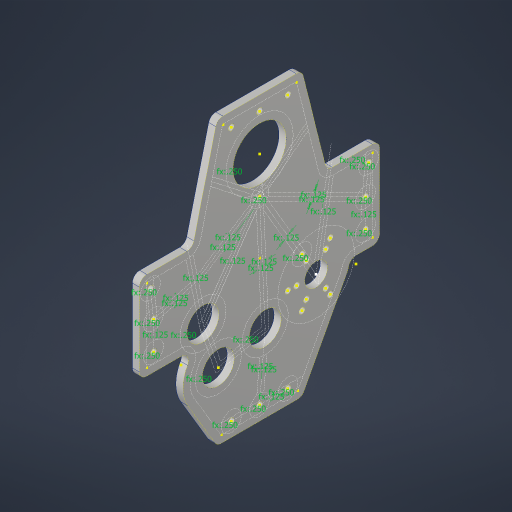
# Autodesk Inventor part: EL2-CGB-001
Saved by Autodesk Inventor 2023.4 (Build 274418000, 418)
## iProperties
Created: 2025-01-19
Part Number: EL2-CGB-001
Material: Aluminum 6061
Document SubType Name: Modeling
Designer: mavericks
Density: 2.7 g/cm^3
Appearance: Aluminum - Flat
Author: mavericks
Autodesk Inventor part; units mm, degrees
ref_plane "YZ Plane" through (0, 0, 0) normal (1, 0, 0) x (0, 1, 0)
ref_plane "XZ Plane" through (0, 0, 0) normal (0, 1, 0) x (-1, 0, 0)
ref_plane "XY Plane" through (0, 0, 0) normal (0, 0, 1) x (1, 0, 0)
sketch "Sketch1" plane through (0, 0, 0) normal (1, 0, 0) x (0, 1, 0)
  line L0 (127, 107.95) -> (-127, 107.95) construction
  line L1 (-127, 107.95) -> (-127, 82.55) construction
  line L2 (-127, 82.55) -> (127, 82.55) construction
  line L3 (127, 82.55) -> (127, 107.95) construction
  line L4 (-44.45, 128.7526) -> (-69.85, 128.7526) construction
  line L5 (-69.85, 128.7526) -> (-69.85, 79.4258) construction
  line L6 (-69.85, 79.4258) -> (-44.45, 79.4258) construction
  line L7 (-44.45, 79.4258) -> (-44.45, 128.7526) construction
  line L8 (69.85, 128.7526) -> (44.45, 128.7526) construction
  line L9 (44.45, 128.7526) -> (44.45, 79.4258) construction
  line L10 (44.45, 79.4258) -> (69.85, 79.4258) construction
  line L11 (69.85, 79.4258) -> (69.85, 128.7526) construction
  line L12 (44.45, 104.0892) -> (-44.45, 104.0892) construction
  line L13 (0, 0) -> (-27.2932, 0) construction
  line L14 (127, -107.95) -> (-127, -107.95) construction
  line L15 (-127, -107.95) -> (-127, -82.55) construction
  line L16 (-127, -82.55) -> (127, -82.55) construction
  line L17 (127, -82.55) -> (127, -107.95) construction
  line L18 (-44.45, -128.7526) -> (-69.85, -128.7526) construction
  line L19 (-69.85, -128.7526) -> (-69.85, -79.4258) construction
  line L20 (-69.85, -79.4258) -> (-44.45, -79.4258) construction
  line L21 (-44.45, -79.4258) -> (-44.45, -128.7526) construction
  line L22 (69.85, -128.7526) -> (44.45, -128.7526) construction
  line L23 (44.45, -128.7526) -> (44.45, -79.4258) construction
  line L24 (44.45, -79.4258) -> (69.85, -79.4258) construction
  line L25 (69.85, -79.4258) -> (69.85, -128.7526) construction
  line L26 (44.45, -104.0892) -> (-44.45, -104.0892) construction
  line L27 (127, 82.55) -> (101.6, 82.55) construction
  line L28 (101.6, 82.55) -> (101.6, -82.55) construction
  line L29 (101.6, -82.55) -> (127, -82.55) construction
  line L30 (127, -82.55) -> (127, 82.55) construction
  line L31 (-127, 82.55) -> (-101.6, 82.55) construction
  line L32 (-101.6, 82.55) -> (-101.6, -82.55) construction
  line L33 (-101.6, -82.55) -> (-127, -82.55) construction
  line L34 (-127, -82.55) -> (-127, 82.55) construction
  point P0 (0, 82.55)
  point P1 (0, 104.0892)
  point P2 (0, -82.55)
  point P3 (0, -104.0892)
  dimension "d0" = 254
  dimension "d1" = 25.4
  dimension "d2" = 82.55
  dimension "d3" = 25.4
  dimension "d4" = 49.3268
  dimension "d6" = 88.9
  dimension "d7" = 3.1242
  dimension "d8" = 25.4
  dimension "d9" = 25.4
  constraints: 70 end point, 16 symmetric about line, 12 parallel, 7 horizontal, 5 perpendicular, 4 midpoint, 2 vertical alignment, 1 horizontal alignment, 1 point on line
  measures "d0" distance of L2.end L1.end
  measures "d1" distance of L1.end L0.end
  measures "d2" vertical distance of L13.start L2.end
  measures "d3" distance of L6.end L5.end
  measures "d4" distance of L5.end L4.end
  measures "d6" distance of L4.start L8.end
  measures "d7" distance from line of L2 L6.end
  measures "d8" distance between parallel lines of L28 L30
  measures "d9" distance between parallel lines of L34 L32
sketch "Sketch2" plane through (0, 0, 0) normal (1, 0, 0) x (0, 1, 0)
  line L0 (-127, 107.95) -> (-127, 82.55) construction
  line L1 (44.45, 104.0892) -> (-44.45, 104.0892) construction
  line L2 (-127, 82.55) -> (127, 82.55) construction
  line L3 (127, 107.95) -> (-127, 107.95) construction
  line L4 (44.45, 79.4258) -> (69.85, 79.4258) construction
  line L5 (127, 82.55) -> (127, 107.95) construction
  line L6 (-69.85, 79.4258) -> (-44.45, 79.4258) construction
  line L7 (-44.45, 79.4258) -> (-44.45, 128.7526) construction
  line L8 (-69.85, 128.7526) -> (-69.85, 79.4258) construction
  line L9 (-44.45, 128.7526) -> (-69.85, 128.7526) construction
  line L10 (101.6, 82.55) -> (101.6, -82.55) construction
  line L11 (127, -82.55) -> (127, 82.55) construction
  line L12 (-127, -82.55) -> (127, -82.55) construction
  line L13 (127, -107.95) -> (-127, -107.95) construction
  line L14 (44.45, -104.0892) -> (-44.45, -104.0892) construction
  line L15 (-127, 82.55) -> (-101.6, 82.55) construction
  line L16 (-101.6, 82.55) -> (-101.6, -82.55) construction
  line L17 (-127, -82.55) -> (-127, 82.55) construction
  line L18 (-69.85, -79.4258) -> (-44.45, -79.4258) construction
  line L19 (-101.6, -82.55) -> (-127, -82.55) construction
  line L20 (-44.45, -79.4258) -> (-44.45, -128.7526) construction
  line L21 (-44.45, -128.7526) -> (-69.85, -128.7526) construction
  line L22 (-69.85, -128.7526) -> (-69.85, -79.4258) construction
  line L23 (-127, -107.95) -> (-127, -82.55) construction
  line L24 (44.45, -79.4258) -> (69.85, -79.4258) construction
  line L25 (44.45, -128.7526) -> (44.45, -79.4258) construction
  line L26 (101.6, -82.55) -> (127, -82.55) construction
  line L27 (69.85, -128.7526) -> (44.45, -128.7526) construction
  line L28 (69.85, -79.4258) -> (69.85, -128.7526) construction
  line L29 (127, -82.55) -> (127, -107.95) construction
  line L30 (69.85, 128.7526) -> (44.45, 128.7526) construction
  line L31 (44.45, 128.7526) -> (44.45, 79.4258) construction
  line L32 (69.85, 79.4258) -> (69.85, 128.7526) construction
  line L33 (127, 82.55) -> (101.6, 82.55) construction
  circle A0 centre (-38.1, -50.8) radius 7.62 construction
  circle A1 centre (-57.15, -5.08) radius 41.91 construction
  circle A2 centre (-57.15, -5.08) radius 11.43 construction
  circle A3 centre (-66.675, 37.0363) radius 31.75 construction
  circle A4 centre (-66.675, 37.0363) radius 15.24 construction
  circle A5 centre (-25.7473, 50.8) radius 27.94 construction
  circle A6 centre (-38.1, -50.8) radius 30.48 construction
  circle A7 centre (-38.1, -50.8) radius 10.16
  circle A8 centre (-57.15, -5.08) radius 14.2875
  circle A9 centre (-66.675, 37.0363) radius 14.2875
  circle A10 centre (-25.7473, 50.8) radius 14.2875
  circle A11 centre (-25.7473, 50.8) radius 20.6375 construction
  circle A12 centre (-66.675, 37.0363) radius 20.6375 construction
  circle A13 centre (-57.15, -5.08) radius 20.6375 construction
  circle A14 centre (-38.1, -50.8) radius 17.4625 construction
  circle A15 centre (-38.1, -50.8) radius 25.4 construction
  line L34 (-41.275, -131.9276) -> (-41.275, -76.2508) construction
  line L35 (-41.275, -76.2508) -> (-73.025, -76.2508) construction
  line L36 (-73.025, -76.2508) -> (-73.025, -131.9276) construction
  line L37 (-73.025, -131.9276) -> (-41.275, -131.9276) construction
  line L38 (-52.3959, -77.7195) -> (-127, -38.1)
  line L39 (-127, -38.1) -> (-127, 38.1)
  line L40 (-127, 38.1) -> (-41.275, 38.1) construction
  line L41 (-41.275, 38.1) -> (-41.275, 104.0892) construction
  arc A16 (-52.3959, -77.7195) -> (-41.275, -81.1142) centre (-38.1, -50.8) ccw
  circle A17 centre (80.9686, 0) radius 23.8125
  circle A18 centre (80.9686, 0) radius 33.3375 construction
  line L42 (37.9487, 60.325) -> (127, 38.1)
  line L43 (127, 38.1) -> (127, -38.1)
  line L44 (127, -38.1) -> (37.9487, -60.325)
  line L45 (37.9487, -60.325) -> (37.9487, -107.95)
  line L46 (37.9487, -107.95) -> (-41.275, -107.95)
  line L47 (-41.275, -107.95) -> (-41.275, -81.1142)
  line L48 (37.9487, 60.325) -> (37.9487, 107.95)
  line L49 (37.9487, 107.95) -> (-41.275, 107.95)
  arc A19 (-23.3654, 68.8297) -> (-38.2397, 37.5831) centre (-25.7473, 50.8) ccw construction
  arc A20 (43.4827, -39.6598) -> (88.1161, 54.1018) centre (80.9686, 0) ccw construction
  line L50 (-41.275, 107.95) -> (-41.275, 56.0863)
  line L51 (-82.9044, 64.325) -> (-127, 38.1)
  arc A21 (-41.275, 56.0863) -> (-82.9044, 64.325) centre (-66.675, 37.0363) ccw
  line L52 (88.1161, 54.1018) -> (-23.3654, 68.8297) construction
  line L53 (43.4827, -39.6598) -> (-38.2397, 37.5831) construction
  circle A22 centre (80.9686, 0) radius 11.1125 construction
  point P0 (25.2487, 98.0186)
  point P1 (0, 95.25)
  point P2 (25.2487, -98.0186)
  point P3 (0, -95.25)
  point P4 (-25.4, -95.25)
  point P5 (-25.4, 95.25)
  point P6 (127, -95.25)
  point P7 (127, 95.25)
  point P8 (0, -82.55)
  point P9 (-114.3, 25.4)
  point P10 (-114.3, 0)
  point P11 (-114.3, -25.4)
  point P12 (-101.6, 0)
  point P13 (-114.3, 82.55)
  point P14 (-38.1, -25.4)
  point P15 (-38.1, -33.3375)
  point P16 (-60.097, -38.1)
  point P17 (-53.223, -42.0688)
  point P18 (-60.097, -63.5)
  point P19 (-53.223, -59.5312)
  point P20 (-38.1, -76.2)
  point P21 (-38.1, -68.2625)
  point P22 (-16.103, -63.5)
  point P23 (-22.977, -59.5313)
  point P24 (-16.103, -38.1)
  point P25 (-22.977, -42.0688)
  point P26 (44.45, 104.0892)
  point P27 (-127, 0)
  point P28 (-127, 0)
  point P29 (101.6, 0)
  point P30 (114.3, 25.4)
  point P31 (114.3, 0)
  point P32 (114.3, -25.4)
  point P33 (114.3, 82.55)
  point P34 (127, 0)
  point P35 (-41.275, -76.8809)
  dimension "d33" = 34.925
  dimension "d34" = 50.8
  dimension "ChainLinks" = 50
  dimension "d10" = 15.24
  dimension "d11" = 83.82
  dimension "d12" = 22.86
  dimension "d13" = 63.5
  dimension "d14" = 30.48
  dimension "d15" = 55.88
  dimension "d16" = 60.96
  dimension "d19" = 63.5
  dimension "d23" = 20.32
  dimension "d24" = 28.575
  dimension "d26" = 25.4
  dimension "d27" = 25.4
  dimension "d28" = 25.4
  dimension "d29" = 25.4
  dimension "d30" = 6.35
  dimension "d31" = 6.35
  dimension "d32" = 6.35
  dimension "d37" = 360
  dimension "d41" = 3.175
  dimension "d42" = 76.2
  dimension "d60" = 101.7513
  dimension "d63" = 31.75
  dimension "d64" = 44.45
  dimension "d66" = 34.925
  dimension "d67" = 31.75
  dimension "d68" = 47.625
  dimension "d70" = 9.525
  dimension "d71" = 47.625
  dimension "d73" = 118.1903
  dimension "d74" = 12.7
  dimension "d75" = 36.3728
  dimension "d76" = 109.1438
  dimension "d78" = 9.9314
  dimension "d79" = 9.9314
  dimension "d133" = 205.5979
  dimension "d134" = 45.7518
  dimension "d135" = 112.4501
  dimension "d141" = 22.225
  constraints: 40 end point, 21 centre point, 18 vertical alignment, 15 coincident, 12 point on circle, 11 horizontal alignment, 11 midpoint, 11 point on line, 9 tangent, 3 collinear, 2 equal radius, 2 perpendicular, 1 horizontal, 1 vertical, 20 other
  measures "d10" diameter of A0
  measures "d11" diameter of A1
  measures "d12" diameter of A2
  measures "d13" diameter of A3
  measures "d14" diameter of A4
  measures "d15" diameter of A5
  measures "d16" diameter of A6
  measures "d19" distance from line of L16 A0.centre
  measures "d23" diameter of A7
  measures "d24" diameter of A8
  measures "d26" distance of point (-25.4, 95.25) point (0, 95.25)
  measures "d27" distance of point (25.249, 98.019) point (0, 95.25)
  measures "d28" distance of point (-114.3, 0) point (-114.3, 25.4)
  measures "d29" distance of point (-114.3, 0) point (-114.3, -25.4)
  measures "d30" radial gap between concentric circles of A10 A11
  measures "d31" radial gap between concentric circles of A9 A12
  measures "d32" radial gap between concentric circles of A8 A13
  measures "d41" distance between parallel lines of L20 L34
  measures "d42" distance of L38.end L39.end
  measures "d60" distance from line of L5 point (25.249, 98.019)
  measures "d63" distance from line of L12 A0.centre
  measures "d64" distance from line of L16 A1.centre
  measures "d66" distance from line of L16 A3.centre
  measures "d67" distance from line of L2 A5.centre
  measures "d68" diameter of A17
  measures "d70" radial gap between concentric circles of A17 A18
  measures "d71" distance of L42.start L48.end
  measures "d73" distance of A17.centre A5.centre
  measures "d74" horizontal distance of point (25.249, 98.019) L48.end
  measures "d75" diameter of A19
  measures "d76" diameter of A20
  measures "d78" distance from line of point (25.249, 98.019) L3
  measures "d79" distance from line of L13 point (25.249, -98.019)
  measures "d135" distance of L52.start L52.end
  measures "d141" diameter of A22
extrude "Extrusion1" add sketch "Sketch2" along normal blind 6.35
hole "Mount Holes" at (0, -101.6, 82.55) at (0, -127, 107.95) at (0, -69.85, 79.4258) at (0, 44.45, -79.4258) at (0, 69.85, -79.4258) at (0, 44.45, -128.7526) at (0, 44.45, 128.7526) at (0, 25.2487, 98.0186) at (0, 0, 95.25) at (0, 25.2487, -98.0186) at (0, 0, -95.25) at (0, -25.4, -95.25) at (0, -25.4, 95.25) at (0, -114.3, 25.4) at (0, -114.3, 0) at (0, -114.3, -25.4) at (0, 114.3, 25.4) at (0, 114.3, 0) at (0, 114.3, -25.4) direction (1, 0, 0) diameter 5.1054 end through all clearance for "Flat Head Machine Screw (82)" size "#10" standard "Ansi Unified Screw Threads"
hole "Motor Mount Holes" at (0, -38.1, -33.3375) at (0, -60.097, -38.1) at (0, -53.223, -42.0688) at (0, -60.097, -63.5) at (0, -53.223, -59.5312) at (0, -16.103, -63.5) at (0, -22.977, -59.5313) at (0, -16.103, -38.1) at (0, -22.977, -42.0688) at (0, -38.1, -25.4) direction (1, 0, 0) diameter 5.1054 end through all clearance for "Flat Head Machine Screw (82)" size "#10" standard "Ansi Unified Screw Threads"
fillet "Fillet1" radius 6.604 12 edges at (3.175, -41.275, 107.95) (3.175, -127, 38.1) (3.175, -127, -38.1) (3.175, -41.275, -81.1142) (3.175, -41.275, -107.95) (3.175, 37.9487, -107.95) (3.175, 37.9487, -60.325) (3.175, 127, -38.1) (3.175, 127, 38.1) (3.175, 37.9487, 60.325) (3.175, 37.9487, 107.95) (3.175, -41.275, 56.0863)
sketch "Sketch8" plane through (6.35, 0, 0) normal (1, 0, 0) x (0, 0, -1)
  arc A0 (-107.95, -34.671) -> (-101.346, -41.275) centre (-101.346, -34.671) ccw projected
  line L0 (-107.95, -34.671) -> (-107.95, 31.3447) projected
  arc A1 (-101.346, 37.9487) -> (-107.95, 31.3447) centre (-101.346, 31.3447) ccw projected
  line L1 (-101.346, 37.9487) -> (-65.4834, 37.9487) projected
  arc A2 (-65.4834, 37.9487) -> (-59.0759, 42.9535) centre (-65.4834, 44.5527) ccw projected
  line L2 (-59.0759, 42.9535) -> (-39.3491, 121.9951) projected
  arc A3 (-32.9416, 127) -> (-39.3491, 121.9951) centre (-32.9416, 120.396) ccw projected
  line L3 (-32.9416, 127) -> (32.9416, 127) projected
  arc A4 (39.3491, 121.9951) -> (32.9416, 127) centre (32.9416, 120.396) ccw projected
  line L4 (39.3491, 121.9951) -> (59.0759, 42.9535) projected
  arc A5 (59.0759, 42.9535) -> (65.4834, 37.9487) centre (65.4834, 44.5527) ccw projected
  line L5 (65.4834, 37.9487) -> (101.346, 37.9487) projected
  arc A6 (107.95, 31.3447) -> (101.346, 37.9487) centre (101.346, 31.3447) ccw projected
  line L6 (107.95, 31.3447) -> (107.95, -34.671) projected
  arc A7 (101.346, -41.275) -> (107.95, -34.671) centre (101.346, -34.671) ccw projected
  line L7 (101.346, -41.275) -> (86.5714, -41.275) projected
  arc A8 (86.5714, -41.275) -> (80.2012, -46.1375) centre (86.5714, -47.879) ccw projected
  arc A9 (77.7195, -52.3959) -> (80.2012, -46.1375) centre (50.8, -38.1) ccw projected
  line L8 (77.7195, -52.3959) -> (39.9622, -123.4934) projected
  arc A10 (34.1297, -127) -> (39.9622, -123.4934) centre (34.1297, -120.396) ccw projected
  line L9 (34.1297, -127) -> (-34.3439, -127) projected
  arc A11 (-40.02, -123.7717) -> (-34.3439, -127) centre (-34.3439, -120.396) ccw projected
  line L10 (-40.02, -123.7717) -> (-64.325, -82.9044) projected
  arc A12 (-64.7124, -51.1154) -> (-64.325, -82.9044) centre (-37.0363, -66.675) ccw projected
  arc A13 (-64.7124, -51.1154) -> (-70.469, -41.275) centre (-70.469, -47.879) ccw projected
  line L11 (-70.469, -41.275) -> (-101.346, -41.275) projected
  circle A14 centre (42.0688, -22.977) radius 2.5527 projected
  circle A15 centre (59.5313, -22.977) radius 2.5527 projected
  circle A16 centre (59.5312, -53.223) radius 2.5527 projected
  circle A17 centre (42.0688, -53.223) radius 2.5527 projected
  circle A18 centre (33.3375, -38.1) radius 2.5527 projected
  circle A19 centre (38.1, -60.097) radius 2.5527 projected
  circle A20 centre (63.5, -60.097) radius 2.5527 projected
  circle A21 centre (63.5, -16.103) radius 2.5527 projected
  circle A22 centre (38.1, -16.103) radius 2.5527 projected
  circle A23 centre (25.4, -38.1) radius 2.5527 projected
  circle A24 centre (0, 114.3) radius 2.5527 projected
  circle A25 centre (25.4, -114.3) radius 2.5527 projected
  circle A26 centre (-25.4, -114.3) radius 2.5527 projected
  circle A27 centre (95.25, -25.4) radius 2.5527 projected
  circle A28 centre (98.0186, 25.2487) radius 2.5527 projected
  circle A29 centre (-98.0186, 25.2487) radius 2.5527 projected
  circle A30 centre (-95.25, 0) radius 2.5527 projected
  circle A31 centre (95.25, 0) radius 2.5527 projected
  circle A32 centre (-95.25, -25.4) radius 2.5527 projected
  circle A33 centre (0, -114.3) radius 2.5527 projected
  circle A34 centre (-25.4, 114.3) radius 2.5527 projected
  circle A35 centre (25.4, 114.3) radius 2.5527 projected
  circle A36 centre (0, 80.9686) radius 23.8125 projected
  circle A37 centre (-50.8, -25.7473) radius 14.2875 projected
  circle A38 centre (-37.0363, -66.675) radius 14.2875 projected
  circle A39 centre (5.08, -57.15) radius 14.2875 projected
  circle A40 centre (50.8, -38.1) radius 10.16 projected
  line L12 (0, 114.3) -> (0, 47.6504) construction
  point P0 (0, 0)
  dimension "d162" = 66.6496
  constraints: 2 end point, 1 vertical, 1 vertical alignment
  measures "d162" distance of L12.start L12.end
hole "Hole4" at (6.35, 47.6504, 0) direction (-1, 0, 0) diameter 3.9624 end through all thread size "10-32 UNF" class "2B" standard "ANSI Unified Screw Threads"
sketch "Sketch9" plane through (6.35, 0, 0) normal (1, 0, 0) x (0, 0, -1)
  circle A0 centre (0, 47.6504) radius 1.9812 construction
  arc A1 (-107.95, -34.671) -> (-101.346, -41.275) centre (-101.346, -34.671) ccw construction
  line L0 (-107.95, -34.671) -> (-107.95, 31.3447) construction
  arc A2 (-101.346, 37.9487) -> (-107.95, 31.3447) centre (-101.346, 31.3447) ccw construction
  line L1 (-101.346, 37.9487) -> (-65.4834, 37.9487) construction
  arc A3 (-65.4834, 37.9487) -> (-59.0759, 42.9535) centre (-65.4834, 44.5527) ccw construction
  line L2 (-59.0759, 42.9535) -> (-39.3491, 121.9951) construction
  arc A4 (-32.9416, 127) -> (-39.3491, 121.9951) centre (-32.9416, 120.396) ccw construction
  line L3 (-32.9416, 127) -> (32.9416, 127) construction
  arc A5 (39.3491, 121.9951) -> (32.9416, 127) centre (32.9416, 120.396) ccw construction
  line L4 (39.3491, 121.9951) -> (59.0759, 42.9535) construction
  arc A6 (59.0759, 42.9535) -> (65.4834, 37.9487) centre (65.4834, 44.5527) ccw construction
  line L5 (65.4834, 37.9487) -> (101.346, 37.9487) construction
  arc A7 (107.95, 31.3447) -> (101.346, 37.9487) centre (101.346, 31.3447) ccw construction
  line L6 (107.95, 31.3447) -> (107.95, -34.671) construction
  arc A8 (101.346, -41.275) -> (107.95, -34.671) centre (101.346, -34.671) ccw construction
  line L7 (101.346, -41.275) -> (86.5714, -41.275) construction
  arc A9 (86.5714, -41.275) -> (80.2012, -46.1375) centre (86.5714, -47.879) ccw construction
  arc A10 (77.7195, -52.3959) -> (80.2012, -46.1375) centre (50.8, -38.1) ccw construction
  line L8 (77.7195, -52.3959) -> (39.9622, -123.4934) construction
  arc A11 (34.1297, -127) -> (39.9622, -123.4934) centre (34.1297, -120.396) ccw construction
  line L9 (34.1297, -127) -> (-34.3439, -127) construction
  arc A12 (-40.02, -123.7717) -> (-34.3439, -127) centre (-34.3439, -120.396) ccw construction
  line L10 (-40.02, -123.7717) -> (-64.325, -82.9044) construction
  arc A13 (-64.7124, -51.1154) -> (-64.325, -82.9044) centre (-37.0363, -66.675) ccw construction
  arc A14 (-64.7124, -51.1154) -> (-70.469, -41.275) centre (-70.469, -47.879) ccw construction
  line L11 (-70.469, -41.275) -> (-101.346, -41.275) construction
  circle A15 centre (42.0688, -22.977) radius 2.5527 construction
  circle A16 centre (59.5313, -22.977) radius 2.5527 construction
  circle A17 centre (59.5312, -53.223) radius 2.5527 construction
  circle A18 centre (42.0688, -53.223) radius 2.5527 construction
  circle A19 centre (33.3375, -38.1) radius 2.5527 construction
  circle A20 centre (38.1, -60.097) radius 2.5527 construction
  circle A21 centre (63.5, -60.097) radius 2.5527 construction
  circle A22 centre (63.5, -16.103) radius 2.5527 construction
  circle A23 centre (38.1, -16.103) radius 2.5527 construction
  circle A24 centre (25.4, -38.1) radius 2.5527 construction
  circle A25 centre (0, 114.3) radius 2.5527 construction
  circle A26 centre (25.4, -114.3) radius 2.5527 construction
  circle A27 centre (-25.4, -114.3) radius 2.5527 construction
  circle A28 centre (95.25, -25.4) radius 2.5527 construction
  circle A29 centre (98.0186, 25.2487) radius 2.5527 construction
  circle A30 centre (-98.0186, 25.2487) radius 2.5527 construction
  circle A31 centre (-95.25, 0) radius 2.5527 construction
  circle A32 centre (95.25, 0) radius 2.5527 construction
  circle A33 centre (-95.25, -25.4) radius 2.5527 construction
  circle A34 centre (0, -114.3) radius 2.5527 construction
  circle A35 centre (-25.4, 114.3) radius 2.5527 construction
  circle A36 centre (25.4, 114.3) radius 2.5527 construction
  circle A37 centre (0, 80.9686) radius 23.8125 construction
  circle A38 centre (-50.8, -25.7473) radius 14.2875 construction
  circle A39 centre (-37.0363, -66.675) radius 14.2875 construction
  circle A40 centre (5.08, -57.15) radius 14.2875 construction
  circle A41 centre (50.8, -38.1) radius 10.16 construction
  circle A42 centre (50.8, -38.1) radius 10.16 construction
  circle A43 centre (50.8, -38.1) radius 34.3027 construction
  circle A44 centre (38.1, -16.103) radius 8.9027 construction
  circle A45 centre (5.08, -57.15) radius 20.6375 construction
  circle A46 centre (-37.0363, -66.675) radius 20.6375 construction
  circle A47 centre (-50.8, -25.7473) radius 20.6375 construction
  circle A48 centre (95.25, 0) radius 8.9027 construction
  circle A49 centre (95.25, -25.4) radius 8.9027 construction
  circle A50 centre (98.0186, 25.2487) radius 8.9027 construction
  line L12 (101.346, 31.5987) -> (65.4834, 31.5987) construction
  arc A51 (52.9149, 41.4159) -> (65.4834, 31.5987) centre (65.4834, 44.5527) ccw construction
  line L13 (52.9149, 41.4159) -> (33.1881, 120.4575) construction
  arc A52 (33.1881, 120.4575) -> (32.9416, 120.65) centre (32.9416, 120.396) ccw construction
  line L14 (32.9416, 120.65) -> (-32.9416, 120.65) construction
  arc A53 (-32.9416, 120.65) -> (-33.1881, 120.4575) centre (-32.9416, 120.396) ccw construction
  line L15 (-33.1881, 120.4575) -> (-52.9149, 41.4159) construction
  arc A54 (-65.4834, 31.5987) -> (-52.9149, 41.4159) centre (-65.4834, 44.5527) ccw construction
  line L16 (-65.4834, 31.5987) -> (-101.346, 31.5987) construction
  arc A55 (-101.346, 31.5987) -> (-101.6, 31.3447) centre (-101.346, 31.3447) ccw construction
  line L17 (-101.6, 31.3447) -> (-101.6, -34.671) construction
  arc A56 (-101.6, -34.671) -> (-101.346, -34.925) centre (-101.346, -34.671) ccw construction
  line L18 (-101.346, -34.925) -> (-70.469, -34.925) construction
  arc A57 (-59.1772, -54.2273) -> (-70.469, -34.925) centre (-70.469, -47.879) ccw construction
  arc A58 (-59.1772, -54.2273) -> (-58.8673, -79.6585) centre (-37.0363, -66.675) ccw construction
  line L19 (-58.8673, -79.6585) -> (-34.5622, -120.5258) construction
  arc A59 (-34.5622, -120.5258) -> (-34.3439, -120.65) centre (-34.3439, -120.396) ccw construction
  line L20 (-34.3439, -120.65) -> (34.1297, -120.65) construction
  arc A60 (34.1297, -120.65) -> (34.354, -120.5151) centre (34.1297, -120.396) ccw construction
  line L21 (34.354, -120.5151) -> (72.1112, -49.4176) construction
  arc A61 (72.1112, -49.4176) -> (74.0759, -44.463) centre (50.8, -38.1) ccw construction
  arc A62 (86.5714, -34.925) -> (74.0759, -44.463) centre (86.5714, -47.879) ccw construction
  line L22 (86.5714, -34.925) -> (101.346, -34.925) construction
  arc A63 (101.346, -34.925) -> (101.6, -34.671) centre (101.346, -34.671) ccw construction
  line L23 (101.6, -34.671) -> (101.6, 31.3447) construction
  arc A64 (101.6, 31.3447) -> (101.346, 31.5987) centre (101.346, 31.3447) ccw construction
  circle A65 centre (0, 80.9686) radius 30.1625 construction
  circle A66 centre (0, 47.6504) radius 8.3312 construction
  circle A67 centre (-98.0186, 25.2487) radius 8.9027 construction
  circle A68 centre (-95.25, 0) radius 8.9027 construction
  circle A69 centre (-95.25, -25.4) radius 8.9027 construction
  circle A70 centre (-25.4, -114.3) radius 8.9027 construction
  circle A71 centre (0, -114.3) radius 8.9027 construction
  circle A72 centre (25.4, -114.3) radius 8.9027 construction
  circle A73 centre (0, 47.6504) radius 1.9812 construction
  line L24 (0, 47.6504) -> (5.08, -57.15) construction
  line L25 (5.08, -57.15) -> (-37.0363, -66.675) construction
  line L26 (-37.0363, -66.675) -> (-50.8, -25.7473) construction
  circle A74 centre (95.25, -25.4) radius 2.5527 construction
  circle A75 centre (95.25, 0) radius 2.5527 construction
  line L27 (95.25, -25.4) -> (95.25, 0) construction
  circle A76 centre (98.0186, 25.2487) radius 2.5527 construction
  line L28 (95.25, 0) -> (98.0186, 25.2487) construction
  line L29 (65.4834, 44.5527) -> (50.8, -38.1) construction
  line L30 (0, 47.6504) -> (95.25, 0) construction
  line L31 (50.8, -38.1) -> (0, 47.6504) construction
  line L32 (-50.8, -25.7473) -> (0, 47.6504) construction
  line L33 (-65.4834, 44.5527) -> (-50.8, -25.7473) construction
  line L34 (0, 47.6504) -> (-43.0515, 80.9367) construction
  line L35 (0, 47.6504) -> (43.0515, 80.9367) construction
  circle A77 centre (-25.4, -114.3) radius 2.5527 construction
  circle A78 centre (0, -114.3) radius 2.5527 construction
  line L36 (-25.4, -114.3) -> (0, -114.3) construction
  circle A79 centre (25.4, -114.3) radius 2.5527 construction
  line L37 (0, -114.3) -> (25.4, -114.3) construction
  line L38 (0, -114.3) -> (5.08, -57.15) construction
  line L39 (-42.2119, 84.3009) -> (4.3247, 48.32) construction
  line L40 (4.3247, 48.32) -> (-52.3965, -33.6329) construction
  line L41 (-52.3965, -33.6329) -> (-66.0212, 31.5987) construction
  line L42 (-43.8911, 77.5725) -> (-2.4223, 45.5099) construction
  line L43 (-2.4223, 45.5099) -> (52.4294, -47.0798) construction
  line L44 (52.4294, -47.0798) -> (66.4068, 31.5987) construction
  line L45 (95.7691, 33.8625) -> (92.5911, 4.8803) construction
  line L46 (92.5911, 4.8803) -> (5.9394, 48.2293) construction
  line L47 (5.9394, 48.2293) -> (43.8911, 77.5725) construction
  line L48 (100.2681, 16.6348) -> (97.9089, -4.8803) construction
  line L49 (97.9089, -4.8803) -> (-5.9394, 47.0715) construction
  line L50 (-5.9394, 47.0715) -> (42.2119, 84.3009) construction
  line L51 (8.3803, -59.6588) -> (2.7179, 57.1563) construction
  line L52 (2.7179, 57.1563) -> (-54.317, -25.2499) construction
  line L53 (-54.317, -25.2499) -> (-39.132, -70.4041) construction
  line L54 (-39.132, -70.4041) -> (8.3803, -59.6588) construction
  line L55 (1.7797, -54.6412) -> (-2.7179, 38.1445) construction
  line L56 (-2.7179, 38.1445) -> (-47.283, -26.2448) construction
  line L57 (-47.283, -26.2448) -> (-34.9407, -62.9459) construction
  line L58 (-34.9407, -62.9459) -> (1.7797, -54.6412) construction
  line L59 (92.075, -17.0827) -> (92.075, 0.1736) construction
  line L60 (92.075, 0.1736) -> (95.7691, 33.8625) construction
  line L61 (64.554, 57.4733) -> (49.1706, -29.1202) construction
  line L62 (49.1706, -29.1202) -> (2.4223, 49.7909) construction
  line L63 (2.4223, 49.7909) -> (-42.2119, 84.3009) construction
  line L64 (-59.8077, 32.9082) -> (-49.2035, -17.8617) construction
  line L65 (-49.2035, -17.8617) -> (-4.3247, 46.9808) construction
  line L66 (-4.3247, 46.9808) -> (-43.8911, 77.5725) construction
  line L67 (6.437, -77.7428) -> (3.8989, -106.2965) construction
  line L68 (-2.4261, -105.7343) -> (0.112, -77.1806) construction
  line L69 (-40.1532, -111.125) -> (39.3407, -111.125) construction
  circle A80 centre (-95.25, -25.4) radius 2.5527 construction
  circle A81 centre (-95.25, 0) radius 2.5527 construction
  line L70 (-95.25, -25.4) -> (-95.25, 0) construction
  line L71 (-95.25, 0) -> (-98.0186, 25.2487) construction
  line L72 (-95.25, 0) -> (-58.1417, 9.4027) construction
  line L73 (-61.8719, 11.7328) -> (-92.4918, 3.9742) construction
  line L74 (-92.4918, 3.9742) -> (-95.7691, 33.8625) construction
  line L75 (-60.5724, 5.5114) -> (-98.0082, -3.9742) construction
  line L76 (-98.0082, -3.9742) -> (-102.0813, 33.1703) construction
  line L77 (-92.075, -17.0827) -> (-92.075, 0.1736) construction
  line L78 (-92.075, 0.1736) -> (-95.7691, 33.8625) construction
  line L79 (-58.1417, 9.4027) -> (0, 47.6504) construction
  line L80 (-8.1799, 46.0698) -> (-55.9879, 14.6199) construction
  line L81 (-54.5921, 7.9373) -> (-4.69, 40.7647) construction
  point P0 (0, 0)
  dimension "d170" = 6.35
  dimension "d171" = 6.35
  dimension "d172" = 6.35
  dimension "d173" = 6.35
  dimension "d174" = 6.35
  dimension "d175" = 6.35
  dimension "d176" = 6.35
  dimension "d177" = 6.35
  dimension "d178" = 6.35
  dimension "d179" = 6.35
  dimension "d180" = 6.35
  dimension "d181" = 6.35
  dimension "d182" = 6.35
  dimension "d183" = 6.35
  dimension "d184" = 6.35
  dimension "d185" = 6.35
  dimension "d186" = 3.175
  dimension "d187" = 3.175
  dimension "d188" = 3.175
  dimension "d189" = 3.175
  dimension "d190" = 3.175
  dimension "d191" = 3.175
  dimension "d192" = 3.175
  dimension "d193" = 3.175
  dimension "d194" = 3.175
  dimension "d195" = 3.175
  dimension "d196" = 3.175
  dimension "d197" = 3.175
  dimension "d198" = 3.175
  dimension "d199" = 3.175
  dimension "d200" = 3.175
  dimension "d201" = 3.175
  dimension "d202" = 3.175
  constraints: 140 end point, 42 point on circle, 28 centre point, 14 point on line, 5 parallel, 3 midpoint, 2 vertical, 1 coincident, 1 collinear, 1 horizontal, 1 tangent, 53 other
  measures "d170" radial gap between concentric circles of A23 A44
  measures "d171" radial gap between concentric circles of A40 A45
  measures "d172" radial gap between concentric circles of A39 A46
  measures "d173" radial gap between concentric circles of A38 A47
  measures "d174" radial gap between concentric circles of A32 A48
  measures "d176" radial gap between concentric circles of A29 A50
  measures "d177" distance between parallel lines of L5 L12
  measures "d178" radial gap between concentric circles of A37 A65
  measures "d179" radial gap between concentric circles of A0 A66
  measures "d180" radial gap between concentric circles of A30 A67
  measures "d181" radial gap between concentric circles of A31 A68
  measures "d183" radial gap between concentric circles of A27 A70
  measures "d184" radial gap between concentric circles of A34 A71
  measures "d185" radial gap between concentric circles of A26 A72
  measures "d186" distance between parallel lines of L32 L40
  measures "d187" distance between parallel lines of L31 L43
  measures "d188" distance between parallel lines of L30 L46
  measures "d189" distance between parallel lines of L30 L49
  measures "d190" distance between parallel lines of L24 L51
  measures "d191" distance between parallel lines of L24 L55
  measures "d192" distance between parallel lines of L27 L59
  measures "d193" distance between parallel lines of L29 L61
  measures "d194" distance between parallel lines of L33 L64
  measures "d195" distance between parallel lines of L37 L69
  measures "d196" distance between parallel lines of L67 L38
  measures "d197" distance between parallel lines of L68 L38
  measures "d198" distance between parallel lines of L72 L73
  measures "d199" distance between parallel lines of L72 L75
  measures "d200" distance between parallel lines of L70 L77
  measures "d201" distance between parallel lines of L79 L80
  measures "d202" distance between parallel lines of L79 L81
equation "\"ChainLinks\" = 50"
equation "\"off\" = 6.35"
body "Solid1"
